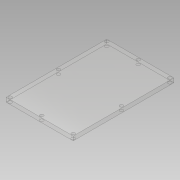
# Autodesk Inventor part: TAPA SUPERIOR
Saved by Autodesk Inventor 2019 (Build 230136000, 136)
## iProperties
Created: 2020-04-08
Part Number: TAPA SUPERIOR
Material: Plástico PMMA
Document SubType Name: Modeling
Designer: Luis Pujol
Density: 1.188 g/cm^3
Appearance: Policarbonato - Claro
Author: Luis Pujol
Autodesk Inventor part; units mm, degrees
ref_plane "YZ Plane" through (0, 0, 0) normal (1, 0, 0) x (0, 1, 0)
ref_plane "XZ Plane" through (0, 0, 0) normal (0, 1, 0) x (-1, 0, 0)
ref_plane "XY Plane" through (0, 0, 0) normal (0, 0, 1) x (1, 0, 0)
sketch "Boceto1" plane through (0, 0, 0) normal (0, 1, 0) x (-1, 0, 0)
  line L0 (-80, 120) -> (80, 120)
  line L1 (80, 120) -> (80, -120)
  line L2 (80, -120) -> (-80, -120)
  line L3 (-80, -120) -> (-80, 120)
  line L4 (-80, 120) -> (80, -120) construction
  line L5 (80, 120) -> (-80, -120) construction
  point P0 (0, 0)
  dimension "d0" = 160
  dimension "d1" = 240
  constraints: 12 end point, 2 midpoint, 2 parallel, 1 horizontal, 1 perpendicular
  measures "d0" distance of L1.end L2.end
  measures "d1" distance of L0.end L1.end
extrude "Extrusión1" add sketch "Boceto1" along normal blind 10
sketch "Boceto2" plane through (0, 10, 0) normal (0, 1, 0) x (1, 0, 0)
  line L0 (-80, -120) -> (80, -120) projected
  line L1 (80, -120) -> (80, 120) projected
  line L2 (80, 120) -> (-80, 120) projected
  line L3 (-80, 120) -> (-80, -120) projected
  line L4 (-75, 115) -> (75, 115) construction
  line L5 (75, 115) -> (75, -115) construction
  line L6 (75, -115) -> (-75, -115) construction
  line L7 (-75, -115) -> (-75, 115) construction
  point P0 (0, 0)
  point P1 (-75, 0)
  point P2 (75, 0)
  point P3 (0, -115)
  point P4 (0, 115)
  dimension "d4" = 5
  constraints: 8 end point, 4 midpoint, 3 other
  measures "d4" distance between parallel lines of L2 L4
hole "Agujero1" at (-75, 10, 0) at (75, 10, 0) at (0, 10, 115) at (0, 10, -115) at (-75, 10, -115) at (75, 10, -115) at (75, 10, 115) at (-75, 10, 115) direction (0, -1, 0) diameter 8 depth 15 tip angle 118
